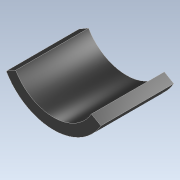
# Autodesk Inventor part: goma
Saved by Autodesk Inventor 2022 (Build 260153000, 153)
## iProperties
Created: 2022-11-16
Part Number: goma
Material: Generic
Document SubType Name: Modeling
Designer: ferna
Density: 1 g/cm^3
Appearance: Glossy - Black
Author: ferna
Autodesk Inventor part; units mm, degrees
ref_plane "YZ Plane" through (0, 0, 0) normal (1, 0, 0) x (0, 1, 0)
ref_plane "XZ Plane" through (0, 0, 0) normal (0, 1, 0) x (-1, 0, 0)
ref_plane "XY Plane" through (0, 0, 0) normal (0, 0, 1) x (1, 0, 0)
sketch "Sketch1" plane through (0, 0, 0) normal (0, 0, 1) x (1, 0, 0)
  arc A0 (-12.9904, -7.5) -> (12.9904, -7.5) centre (0, 0) ccw
  line L0 (0, 0) -> (12.9904, -7.5) construction
  line L1 (0, 0) -> (15, 0) construction
  line L2 (0, 0) -> (-12.9904, -7.5) construction
  arc A1 (-10.3923, -6) -> (10.3923, -6) centre (0, 0) ccw
  line L3 (-12.9904, -7.5) -> (-10.3923, -6)
  line L4 (12.9904, -7.5) -> (10.3923, -6)
  dimension "d0" = 15
  dimension "d1" = 30
  dimension "d2" = 120
  dimension "d3" = 12
  constraints: 10 end point, 4 point on circle, 2 centre point, 2 coincident, 2 collinear, 2 point on line, 1 equal length, 1 horizontal
  measures "d0" radius of A0
  measures "d1" angle of L0 L1
  measures "d2" angle of L2 L0
  measures "d3" radius of A1
extrude "Extrusion1" add sketch "Sketch1" along normal blind 20
body "Solid1"
